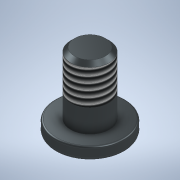
# Autodesk Inventor part: Perno M5x8cabeza plana_
Saved by Autodesk Inventor 2022 (Build 260153000, 153)
## iProperties
Created: 2020-05-08
Part Number: Perno M5x8cabeza plana_
Material: Hierro, gris
Document SubType Name: Modeling
Designer: andre
Density: 7.15 g/cm^3
Appearance: Gris hierro
Author: andre
Autodesk Inventor part; units mm, degrees
ref_plane "YZ Plane" through (0, 0, 0) normal (1, 0, 0) x (0, 1, 0)
ref_plane "XZ Plane" through (0, 0, 0) normal (0, 1, 0) x (-1, 0, 0)
ref_plane "XY Plane" through (0, 0, 0) normal (0, 0, 1) x (1, 0, 0)
sketch "Boceto1" plane through (0, 0, 0) normal (0, 1, 0) x (-1, 0, 0)
  circle A0 centre (0, 0) radius 4.5
  dimension "d0" = 9
  constraints: 1 centre point, 1 coincident
  measures "d0" diameter of A0
extrude "Extrusión1" add sketch "Boceto1" along normal blind 1.6
sketch "Boceto2" plane through (0, 1.6, 0) normal (0, 1, 0) x (1, 0, 0)
  circle A0 centre (0, 0) radius 2.5
  dimension "d3" = 5
  constraints: 1 centre point, 1 coincident
  measures "d3" diameter of A0
extrude "Extrusión2" add sketch "Boceto2" along normal blind 8
fillet "Empalme1" radius 0.4 1 edges at (4.5, 0, 0)
fillet "Empalme2" radius 0.2 1 edges at (4.5, 1.6, 0)
sketch "Boceto3" plane through (0, 0, 0) normal (0, -1, 0) x (1, 0, 0)
  line L0 (-1.7321, 0) -> (-0.866, 1.5)
  line L1 (-0.866, 1.5) -> (0.866, 1.5)
  line L2 (0.866, 1.5) -> (1.7321, 0)
  line L3 (1.7321, 0) -> (0.866, -1.5)
  line L4 (0.866, -1.5) -> (-0.866, -1.5)
  line L5 (-0.866, -1.5) -> (-1.7321, 0)
  point P0 (0, 0)
  point P1 (0, 0)
  dimension "d8" = 3
  constraints: 12 end point, 1 coincident, 13 other
  measures "d8" distance between parallel lines of L1 L4
extrude "Extrusión3" cut sketch "Boceto3" against normal blind 2.5
chamfer "Chaflán1" distance 0.5 angle 45 1 edges at (-2.5, 9.6, 0)
thread "Rosca2" size "M5x0.8" class "6g" standard "ANSI Metric M Profile" length 12 offset 3
